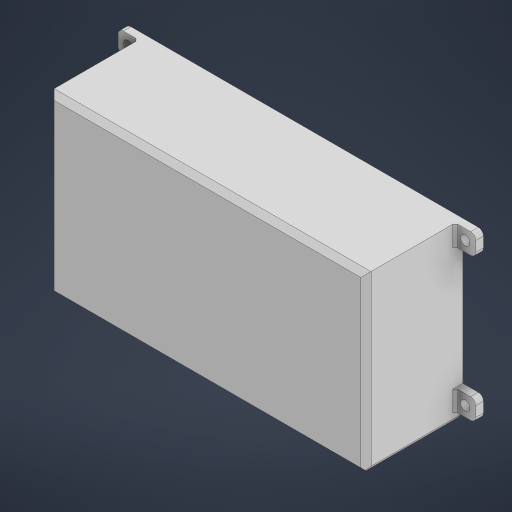
# Autodesk Inventor part: lid
Saved by Autodesk Inventor 2024 (Build 280153000, 153)
## iProperties
Created: 2024-08-05
Part Number: lid
Material: Generic
Document SubType Name: Modeling
Designer: micjo
Density: 1 g/cm^3
Appearance: Default
Author: micjo
Autodesk Inventor part; units mm, degrees
ref_plane "YZ Plane" through (0, 0, 0) normal (1, 0, 0) x (0, 1, 0)
ref_plane "XZ Plane" through (0, 0, 0) normal (0, 1, 0) x (-1, 0, 0)
ref_plane "XY Plane" through (0, 0, 0) normal (0, 0, 1) x (1, 0, 0)
sketch "Sketch1" plane through (0, 0, 0) normal (0, 0, 1) x (1, 0, 0)
  line L0 (-65.9426, 37.0033) -> (-65.9426, 29.0033)
  line L1 (-65.9426, 37.0033) -> (73.8428, 37.0033)
  line L2 (73.8428, 37.0033) -> (73.8428, 29.0033)
  line L3 (66.0574, -18.9471) -> (66.0574, 29.0033)
  line L4 (73.8428, 29.0033) -> (66.0574, 29.0033)
  line L5 (74.0574, -18.9471) -> (66.0574, -18.9471)
  line L6 (66.0574, 29.0033) -> (66.0574, -18.9471)
  line L7 (66.0574, -18.9471) -> (74.0574, -18.9471)
  line L8 (66.0574, -26.9471) -> (74.0574, -26.9471)
  line L9 (74.0574, -18.9471) -> (74.0574, -26.9471)
  line L10 (74.0574, -26.9471) -> (66.0574, -26.9471)
  line L11 (66.0574, -26.9471) -> (66.0574, -28.9967)
  line L12 (-55.9426, -31.4967) -> (64.0574, -31.4967)
  line L13 (66.0574, -28.9967) -> (64.0574, -31.4967)
  line L14 (64.0574, -31.4967) -> (-55.9426, -31.4967)
  line L15 (-55.9426, -31.4967) -> (-57.9426, -28.9967)
  line L16 (-55.9426, -31.4967) -> (-57.9426, -28.9967)
  line L17 (-57.9426, -28.9967) -> (-57.9426, -26.9471)
  line L18 (-57.9426, -26.9471) -> (-65.9823, -26.9471)
  line L19 (-65.9823, -26.9471) -> (-65.9823, -18.9471)
  line L20 (-57.9426, -18.9471) -> (-65.9426, -18.9471)
  line L21 (-65.9823, -18.9471) -> (-57.9426, -18.9471)
  line L22 (-57.9426, -18.9471) -> (-57.9426, 29.0033)
  line L23 (-57.9426, 29.0033) -> (-65.9426, 29.0033)
  line L24 (-55.9426, 35.0033) -> (-28.9426, 35.0033)
  line L25 (62.5574, -26.9967) -> (64.0574, -26.9967)
  line L26 (-55.9426, 35.0033) -> (64.0574, 35.0033)
  line L27 (64.0574, 35.0033) -> (64.0574, -26.9967)
  line L28 (64.0574, -26.9967) -> (-55.9426, -26.9967)
  line L29 (-55.9426, -26.9967) -> (-55.9426, 35.0033)
  point P0 (0, 0)
  constraints: 60 end point, 8 perpendicular, 6 point on line, 4 parallel, 3 collinear, 2 horizontal
extrude "Extrusion1" add sketch "Sketch1" along normal blind 36
sketch "Sketch2" plane through (-55.9426, -31.4967, 0) normal (0, -1, 0) x (1, 0, 0)
  line L0 (120, 0) -> (120, 36) projected
  line L1 (120, 18) -> (0, 18)
  line L2 (0, 0) -> (0, 36) projected
  line L3 (120, 18) -> (85, 18)
  line L4 (71.5, 8) -> (98.5, 8)
  line L5 (98.5, 8) -> (98.5, 28)
  line L6 (98.5, 28) -> (71.5, 28)
  line L7 (71.5, 28) -> (71.5, 8)
  line L8 (71.5, 8) -> (98.5, 28) construction
  line L9 (98.5, 8) -> (71.5, 28) construction
  line L10 (85, 18) -> (65, 18)
  line L11 (85, 18) -> (105, 18)
  circle A0 centre (65, 18) radius 2.4
  circle A1 centre (105, 18) radius 2.4
  point P0 (55.9426, 0)
  dimension "d2" = 35
  dimension "d3" = 27
  dimension "d4" = 20
  dimension "d5" = 20
  dimension "d6" = 20
  dimension "d7" = 4.8
  constraints: 20 end point, 4 midpoint, 3 point on line, 2 centre point, 2 coincident, 2 parallel, 1 equal radius, 1 horizontal, 1 perpendicular
  measures "d2" distance of L1.start L3.end
  measures "d3" distance of L6.end L5.end
  measures "d4" distance of L5.end L4.end
  measures "d5" distance of L3.end L10.end
  measures "d6" distance of L3.end L11.end
  measures "d7" diameter of A0
extrude "Extrusion2" cut sketch "Sketch2" against normal up to surface (4.5 mm away)
chamfer "Chamfer1" distance 5 angle 45 2 edges at (42.5574, -29.2467, 8) (15.5574, -29.2467, 8)
fillet "Fillet1" radius 1.5 6 edges at (15.5574, -29.2467, 13) (20.5574, -29.2467, 8) (37.5574, -29.2467, 8) (42.5574, -29.2467, 13) (42.5574, -29.2467, 28) (15.5574, -29.2467, 28)
sketch "Sketch3" plane through (-55.9426, -31.4967, 0) normal (0, -1, 0) x (1, 0, 0)
  circle A0 centre (65, 18) radius 2.4 projected
  line L0 (65, 18) -> (35, 18)
  line L1 (65, 18) -> (95, 18) construction
  line L2 (19.65, 7) -> (50.35, 7)
  line L3 (50.35, 7) -> (50.35, 29)
  line L4 (50.35, 29) -> (19.65, 29)
  line L5 (19.65, 29) -> (19.65, 7)
  line L6 (19.65, 7) -> (50.35, 29) construction
  line L7 (50.35, 7) -> (19.65, 29) construction
  point P0 (55.9426, 0)
  dimension "d14" = 30
  dimension "d15" = 180
  dimension "d16" = 30.7
  dimension "d17" = 22
  constraints: 16 end point, 3 horizontal, 2 midpoint, 2 parallel, 1 collinear, 1 perpendicular
  measures "d14" distance of L0.start L0.end
  measures "d15" angle of L0 L1
  measures "d16" distance of L4.end L3.end
  measures "d17" distance of L3.end L2.end
extrude "Extrusion3" cut sketch "Sketch3" against normal up to surface (4.5 mm away) contours L5 L4 L3 L2
sketch "Sketch4" plane through (-57.9426, -18.9471, 0) normal (-1, 0, 0) x (0, 0, 1)
  line L0 (0, 47.9504) -> (36, 47.9504) projected
  line L1 (18, 47.9504) -> (18, 0)
  line L2 (0, 0) -> (36, 0) projected
  circle A0 centre (18, 25.0155) radius 3.75
  point P0 (0, 18.9471)
  dimension "d20" = 7.5
  constraints: 2 end point, 2 midpoint, 1 centre point, 1 point on line
  measures "d20" diameter of A0
extrude "Extrusion4" cut sketch "Sketch4" against normal up to surface (2 mm away)
sketch "Sketch5" plane through (0, 0, 36) normal (0, 0, 1) x (1, 0, 0)
  line L0 (73.8428, 37.0033) -> (-65.9426, 37.0033) projected
  line L1 (-65.9426, 37.0033) -> (-57.9426, 37.0033)
  line L2 (-57.9426, 37.0033) -> (-57.9426, 29.0033)
  line L3 (-57.9426, 29.0033) -> (-65.9426, 29.0033)
  line L4 (-65.9426, 29.0033) -> (-65.9426, 37.0033)
  line L5 (-65.9823, -26.9471) -> (-57.9426, -26.9471) projected
  line L6 (-57.9426, -18.9471) -> (-65.9823, -18.9471) projected
  line L7 (-57.9426, -26.9471) -> (-65.9823, -26.9471)
  line L8 (-65.9823, -26.9471) -> (-65.9823, -18.9471)
  line L9 (-65.9823, -18.9471) -> (-57.9426, -18.9471)
  line L10 (-57.9426, -18.9471) -> (-57.9426, -26.9471)
  line L11 (66.0574, -18.9471) -> (66.0574, 29.0033) projected
  line L12 (74.0574, -26.9471) -> (74.0574, -18.9471) projected
  line L13 (66.0574, -18.9471) -> (74.0574, -18.9471)
  line L14 (74.0574, -18.9471) -> (74.0574, -26.9471)
  line L15 (74.0574, -26.9471) -> (66.0574, -26.9471)
  line L16 (66.0574, -26.9471) -> (66.0574, -18.9471)
  line L17 (66.0574, 29.0033) -> (74.0574, 29.0033)
  line L18 (74.0574, 29.0033) -> (74.0574, 37.0033)
  line L19 (74.0574, 37.0033) -> (66.0574, 37.0033)
  line L20 (66.0574, 37.0033) -> (66.0574, 29.0033)
  point P0 (0, 0)
  constraints: 32 end point, 8 parallel, 4 horizontal, 4 perpendicular, 4 point on line
extrude "Extrusion5" cut sketch "Sketch5" against normal blind 33
sketch "Sketch6" plane through (0, 0, 36) normal (0, 0, 1) x (1, 0, 0)
  line L0 (66.0574, 37.0033) -> (-57.9426, 37.0033) projected
  line L1 (-57.9426, 37.0033) -> (66.0574, 37.0033)
  line L2 (66.0574, 37.0033) -> (66.0574, -31.4967)
  line L3 (66.0574, -31.4967) -> (-57.9426, -31.4967)
  line L4 (-57.9426, -31.4967) -> (-57.9426, 37.0033)
  point P0 (0, 0)
  constraints: 8 end point, 2 parallel, 1 horizontal, 1 perpendicular
extrude "Extrusion6" add sketch "Sketch6" along normal blind 2
chamfer "Chamfer2" distance 2 distance2 2.5 1 edges at (66.0574, -31.4967, 37) measured on face at (0.8407, -31.4967, 35)
chamfer "Chamfer3" distance 2.5 distance2 2 1 edges at (-57.9426, -31.4967, 37) measured on face at (-57.9426, 4.6917, 31.9167)
sketch "Sketch7" plane through (0, 0, 36) normal (0, 0, -1) x (-1, 0, 0)
  line L0 (55.9426, -26.9967) -> (55.9426, 35.0033) projected
  line L1 (55.9426, -26.9967) -> (55.9426, -12.9967)
  line L2 (55.9426, 35.0033) -> (-64.0574, 35.0033) projected
  line L3 (55.9426, -12.9967) -> (55.9426, -2.9967)
  line L4 (55.9426, -2.9967) -> (55.9426, 11.0033)
  line L5 (55.9426, 11.0033) -> (55.9426, 21.0033)
  line L6 (55.9426, -12.9967) -> (-64.0574, -12.9967)
  line L7 (-64.0574, -12.9967) -> (-64.0574, -2.9967)
  line L8 (-64.0574, -2.9967) -> (55.9426, -2.9967)
  line L9 (55.9426, -2.9967) -> (55.9426, -12.9967)
  line L10 (55.9426, 11.0033) -> (-64.0574, 11.0033)
  line L11 (-64.0574, 11.0033) -> (-64.0574, 21.0033)
  line L12 (-64.0574, 21.0033) -> (55.9426, 21.0033)
  line L13 (55.9426, 21.0033) -> (55.9426, 11.0033)
  point P0 (0, 0)
  dimension "d33" = 14
  dimension "d34" = 10
  dimension "d35" = 14
  dimension "d36" = 10
  constraints: 24 end point, 4 parallel, 4 point on line, 3 perpendicular, 2 horizontal
  measures "d33" distance of L0.start L1.end
  measures "d34" distance of L1.end L3.end
  measures "d35" distance of L3.end L4.end
  measures "d36" distance of L4.end L5.end
extrude "Extrusion7" add sketch "Sketch7" along normal blind 2
chamfer "Chamfer4" distance 2 angle 45 4 edges at (4.0574, 11.0033, 36) (4.0574, -2.9967, 36) (4.0574, 21.0033, 36) (4.0574, -12.9967, 36)
chamfer "Chamfer5" distance 2 angle 45 4 edges at (-57.9426, 4.0032, 38) (4.0574, 37.0033, 38) (66.0574, 4.0032, 38) (4.0574, -31.4967, 38)
sketch "Sketch8" plane through (0, 0, 3) normal (0, 0, 1) x (1, 0, 0)
  line L0 (-65.9426, 29.0033) -> (-65.9426, 37.0033) projected
  line L1 (-65.9426, 33.0033) -> (73.8428, 33.0033)
  line L2 (-65.9823, -18.9471) -> (-65.9823, -26.9471) projected
  line L3 (-65.9823, -22.9471) -> (74.0574, -22.9471)
  circle A0 centre (-61.9426, 33.0033) radius 1.85
  line L4 (73.8428, 29.0033) -> (66.0574, 29.0033) projected
  circle A1 centre (69.9501, -22.9471) radius 1.85
  circle A2 centre (-61.9426, -22.9471) radius 1.85
  circle A3 centre (69.9501, 33.0033) radius 1.85
  point P0 (0, 0)
  dimension "d45" = 3.7
  constraints: 4 centre point, 4 end point, 4 point on line, 3 equal radius, 2 horizontal, 2 midpoint
  measures "d45" diameter of A0
extrude "Extrusion8" cut sketch "Sketch8" against normal up to surface (3 mm away)
sketch "Sketch10" plane through (-65.9426, 37.0033, 0) normal (0, 1, 0) x (1, 0, 0)
  line L0 (132, -36) -> (132, -3) projected
  line L1 (140, 0) -> (140, -3) projected
  line L2 (132, -3) -> (140, -3)
  line L3 (140, -3) -> (140, 0)
  line L4 (139.7854, 0) -> (139.7854, -3) projected
  line L5 (140, 0) -> (139.7854, 0)
  line L6 (139.7854, 0) -> (139.7854, -3)
  point P0 (65.9426, 0)
  constraints: 8 end point, 2 equal length, 2 perpendicular
extrude "Extrusion10" add sketch "Sketch10" against normal up to surface (8 mm away)
sketch "Sketch12" plane through (0, 0, 38) normal (0, 0, 1) x (1, 0, 0)
  circle A0 centre (-61.9426, 33.0033) radius 1.85 projected
  circle A1 centre (-61.9426, 33.0033) radius 3.25
  circle A2 centre (69.9501, 33.0033) radius 1.85 projected
  circle A3 centre (69.9501, 33.0033) radius 3.25
  circle A4 centre (69.9501, -22.9471) radius 1.85 projected
  circle A5 centre (69.9501, -22.9471) radius 3.25
  circle A6 centre (-61.9426, -22.9471) radius 1.85 projected
  circle A7 centre (-61.9426, -22.9471) radius 3.25
  point P0 (0, 0)
  dimension "d57" = 6.5
  dimension "d58" = 6.5
  dimension "d59" = 6.5
  dimension "d60" = 6.5
  constraints: 4 centre point, 4 coincident
  measures "d57" diameter of A1
  measures "d58" diameter of A3
  measures "d59" diameter of A5
  measures "d60" diameter of A7
extrude "Extrusion12" cut sketch "Sketch12" against normal blind 35 contours A0 | A1 | A2 | A3 | A4 | A5 | A6 | A7
chamfer "Chamfer6" distance 1 angle 45 4 edges at (66.0574, -22.9471, 3) (66.0574, 33.0033, 3) (-57.9426, 33.0033, 3) (-57.9426, -22.9471, 3)
fillet "Fillet3" radius 2 8 edges at (-65.9426, 37.0033, 1.5) (-65.9426, 29.0033, 1.5) (-65.9823, -18.9471, 1.5) (-65.9823, -26.9471, 1.5) (74.0574, 29.0033, 1.5) (74.0574, -18.9471, 1.5) (74.0574, -26.9471, 1.5) (74.0574, 37.0033, 1.5)
body "Solid1"
